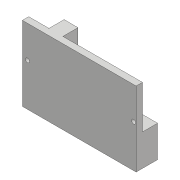
# Autodesk Inventor part: Eth_Switch
Saved by Autodesk Inventor 2018 (Build 220112000, 112)
## iProperties
Created: 2019-09-10
Part Number: Eth_Switch
Material: Generic
Document SubType Name: Modeling
Designer: Clevo
Density: 1 g/cm^3
Appearance: Default
Author: Clevo
Autodesk Inventor part; units mm, degrees
ref_plane "YZ Plane" through (0, 0, 0) normal (1, 0, 0) x (0, 1, 0)
ref_plane "XZ Plane" through (0, 0, 0) normal (0, 1, 0) x (-1, 0, 0)
ref_plane "XY Plane" through (0, 0, 0) normal (0, 0, 1) x (1, 0, 0)
sketch "Sketch1" plane through (0, 0, 0) normal (0, 1, 0) x (-1, 0, 0)
  line L0 (-45, -29.5) -> (45, -29.5)
  line L1 (45, -29.5) -> (45, 29.5)
  line L2 (45, 29.5) -> (-45, 29.5)
  line L3 (-45, 29.5) -> (-45, -29.5)
  line L4 (-45, -29.5) -> (45, 29.5) construction
  line L5 (45, -29.5) -> (-45, 29.5) construction
  point P0 (0, 0)
  dimension "d0" = 59
  dimension "d1" = 90
  constraints: 12 end point, 2 midpoint, 2 parallel, 1 horizontal, 1 perpendicular
  measures "d0" distance of L0.end L1.end
  measures "d1" distance of L1.end L2.end
extrude "Extrusion1" add sketch "Sketch1" along normal blind 17
sketch "Sketch2" plane through (0, 17, 0) normal (0, 1, 0) x (1, 0, 0)
  line L0 (-45, 29.5) -> (-45, -29.5) projected
  line L1 (-45, -29.5) -> (-29, -29.5)
  line L2 (-29, -29.5) -> (-29, 4.5)
  line L3 (-29, 4.5) -> (-45, 4.5)
  line L4 (-45, 4.5) -> (-45, -29.5)
  line L5 (45, -29.5) -> (-18, -29.5)
  line L6 (-18, -29.5) -> (-18, 4.5)
  line L7 (-18, 4.5) -> (45, 4.5)
  line L8 (45, 4.5) -> (45, -29.5)
  line L9 (45, 29.5) -> (-45, 29.5) projected
  line L10 (45, -29.5) -> (45, 29.5) projected
  line L11 (-45, -29.5) -> (45, -29.5) projected
  point P0 (0, 0)
  dimension "d4" = 25
  dimension "d5" = 25
  dimension "d6" = 16
  dimension "d7" = 63
  constraints: 16 end point, 4 parallel, 2 collinear, 2 horizontal, 2 perpendicular
  measures "d4" distance between parallel lines of L9 L7
  measures "d5" distance between parallel lines of L9 L3
  measures "d6" distance of L2.end L3.end
  measures "d7" distance of L6.end L7.end
extrude "Extrusion2" cut sketch "Sketch2" against normal blind 12 contours L3 L2 L1 L0 | L8 L5 L6 L7
sketch "Sketch3" plane through (0, 0, 0) normal (0, -1, 0) x (1, 0, 0)
  line L0 (-41, 4.1) -> (43, 4.1)
  line L1 (-45, -29.5) -> (-45, 29.5) projected
  line L2 (45, 29.5) -> (45, -29.5) projected
  line L3 (-45, 29.5) -> (45, 29.5) projected
  point P0 (0, 0)
  dimension "d10" = 4
  dimension "d11" = 2
  dimension "d12" = 25.4
  constraints: 2 end point, 1 horizontal
  measures "d10" distance from line of L1 L0.start
  measures "d11" distance from line of L2 L0.end
  measures "d12" distance between parallel lines of L3 L0
hole "Hole1" at (-41, 0, 4.1) at (43, 0, 4.1) direction (0, 1, 0) diameter 3.2 end through all clearance for "Flat Head Machine Screw" size "M3" standard "Ansi Metric M Profile"
equation "\"d5\" = d4"
body "Solid1"
